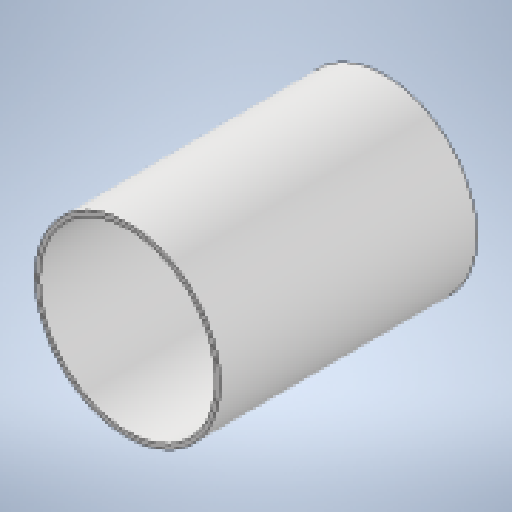
# Autodesk Inventor part: TZS 1221 charging tube
Saved by Autodesk Inventor 2025.1 (Build 291241020, 241B)
## iProperties
Created: 2025-02-12
Part Number: TZS 1221 charging tube
Material: Steel
Document SubType Name: Modeling
Designer: admin
Density: 7.85 g/cm^3
Appearance: Default
Mass: 3580.85 g
Surface Area: 2322.27 cm^2
Volume: 456.159 cm^3
Author: pokla
Autodesk Inventor part; units mm, degrees
ref_plane "YZ Plane" through (0, 0, 0) normal (1, 0, 0) x (0, 1, 0)
ref_plane "XZ Plane" through (0, 0, 0) normal (0, 1, 0) x (-1, 0, 0)
ref_plane "XY Plane" through (0, 0, 0) normal (0, 0, 1) x (1, 0, 0)
sketch "Sketch1" plane through (0, 0, 0) normal (0, 1, 0) x (-1, 0, 0)
  circle A0 centre (0, 0) radius 79.5
  circle A1 centre (0, 0) radius 75.5
  line L0 (79.5, 0) -> (-79.5, 0)
  point P0 (-75.5, 0)
  point P1 (75.5, 0)
  dimension "d0" = 159
  dimension "d1" = 4
  constraints: 3 coincident, 2 centre point, 2 end point, 2 point on circle, 1 horizontal, 1 midpoint
  measures "d0" diameter of A0
  measures "d1" radial gap between concentric circles of A0 A1
extrude "Extrusion1" add sketch "Sketch1" against normal blind 220 contours L0 A1 A0 | A0 L0 A1
body "Solid1"
